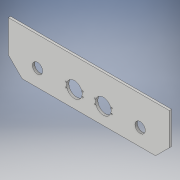
# Autodesk Inventor part: MecanumDriveTrainPlate17-18
Saved by Autodesk Inventor 2017 (Build 210142000, 142)
## iProperties
Created: 2017-09-16
Part Number: MecanumDriveTrainPlate17-18
Material: Generic
Document SubType Name: Modeling
Designer: User
Density: 1 g/cm^3
Appearance: Default
Author: User
Autodesk Inventor part; units mm, degrees
ref_plane "YZ Plane" through (0, 0, 0) normal (1, 0, 0) x (0, 1, 0)
ref_plane "XZ Plane" through (0, 0, 0) normal (0, 1, 0) x (-1, 0, 0)
ref_plane "XY Plane" through (0, 0, 0) normal (0, 0, 1) x (1, 0, 0)
sketch "Sketch1" plane through (0, 0, 0) normal (0, 0, 1) x (1, 0, 0)
  line L0 (0, 0) -> (444.5, 0)
  line L1 (444.5, 0) -> (444.5, 127)
  line L2 (444.5, 127) -> (0, 127)
  line L3 (0, 127) -> (0, 0)
  dimension "d0" = 444.5
  dimension "d1" = 127
  constraints: 8 end point, 2 perpendicular, 1 horizontal, 1 vertical
  measures "d0" distance of L0.start L0.end
  measures "d1" distance of L0.end L1.end
extrude "Extrusion1" add sketch "Sketch1" along normal blind 6.35
sketch "Sketch2" plane through (0, 0, 6.35) normal (0, 0, 1) x (1, 0, 0)
  line L0 (0, 0) -> (444.5, 0) projected
  line L1 (38.0923, 0) -> (0, 38.0919)
  line L2 (0, 127) -> (0, 0) projected
  line L3 (0, 0) -> (444.5, 0) projected
  line L4 (444.5, 0) -> (444.5, 127) projected
  line L5 (444.5, 0) -> (406.4, 0)
  line L6 (444.5, 0) -> (482.6, 0) construction
  line L7 (444.5, 0) -> (444.5, 38.0919)
  line L8 (444.5, 38.0919) -> (406.4086, 0)
  point P0 (419.1126, 0)
  dimension "d19" = 38.1
  dimension "d20" = 180
  constraints: 10 end point, 5 point on line, 3 collinear, 1 horizontal
  measures "d19" distance of L0.end L5.end
  measures "d20" angle of L5 L6
extrude "Extrusion2" cut sketch "Sketch2" against normal blind 50.8
sketch "Sketch3" plane through (0, 0, 6.35) normal (0, 0, 1) x (1, 0, 0)
  line L0 (0, 77.664) -> (80.645, 77.664) construction
  line L1 (444.5, 127) -> (0, 127) projected
  line L2 (80.645, 127) -> (161.29, 127) construction
  circle A0 centre (80.645, 46.355) radius 14.2748
  line L3 (444.5, 38.0919) -> (444.5, 127) projected
  line L4 (444.5, 77.664) -> (525.145, 77.664) construction
  line L5 (444.5, 38.0919) -> (444.5, 127) projected
  line L6 (444.5, 46.355) -> (525.145, 46.355) construction
  circle A1 centre (363.855, 46.355) radius 14.2748
  line L7 (444.5, 127) -> (0, 127) projected
  line L8 (0, 127) -> (0, 38.0919) projected
  circle A2 centre (182.245, 46.355) radius 21.59
  circle A3 centre (262.255, 46.355) radius 21.59
  line L9 (182.245, 46.355) -> (159.131, 46.355)
  line L10 (159.131, 46.355) -> (159.131, 53.3654)
  line L11 (159.131, 53.3654) -> (159.131, 46.355)
  line L12 (159.131, 46.355) -> (159.131, 39.3446)
  circle A4 centre (159.131, 39.3446) radius 1.7526
  circle A5 centre (159.131, 53.3654) radius 1.7526
  line L13 (182.245, 46.355) -> (205.359, 46.355)
  line L14 (205.359, 46.355) -> (205.359, 53.3654)
  line L15 (205.359, 53.3654) -> (205.359, 46.355)
  line L16 (205.359, 46.355) -> (205.359, 39.3446)
  circle A6 centre (205.359, 39.3446) radius 1.7526
  circle A7 centre (205.359, 53.3654) radius 1.7526
  line L17 (262.255, 46.355) -> (239.141, 46.355)
  line L18 (239.141, 46.355) -> (239.141, 53.3654)
  line L19 (239.141, 46.355) -> (239.141, 39.3446)
  circle A8 centre (239.141, 39.3446) radius 1.7526
  circle A9 centre (239.141, 53.3654) radius 1.7526
  line L20 (262.255, 46.355) -> (285.369, 46.355)
  line L21 (285.369, 46.355) -> (285.369, 39.3446)
  line L22 (285.369, 46.355) -> (285.369, 53.3654)
  circle A10 centre (285.369, 53.3654) radius 1.7526
  circle A11 centre (285.369, 39.3446) radius 1.7526
  point P0 (0, 0)
  dimension "d10" = 28.5496
  dimension "d18" = 28.5496
  dimension "d31" = 43.18
  dimension "d32" = 43.18
  dimension "d35" = 23.114
  dimension "d36" = 7.0104
  dimension "d37" = 7.0104
  dimension "d38" = 3.5052
  dimension "d39" = 3.5052
  dimension "d40" = 23.114
  dimension "d41" = 7.0104
  dimension "d42" = 7.0104
  dimension "d43" = 3.5052
  dimension "d44" = 3.5052
  dimension "d45" = 23.114
  dimension "d46" = 3.5052
  dimension "d47" = 3.5052
  dimension "d48" = 23.114
  dimension "d49" = 3.5052
  dimension "d50" = 3.5052
  constraints: 36 end point, 12 centre point, 8 coincident, 8 horizontal, 4 point on line, 4 vertical, 3 perpendicular, 2 collinear
  measures "d10" diameter of A0
  measures "d18" diameter of A1
  measures "d31" diameter of A2
  measures "d32" diameter of A3
  measures "d35" distance of L9.start L9.end
  measures "d36" distance of L9.end L10.end
  measures "d37" distance of L9.end L12.end
  measures "d38" diameter of A4
  measures "d39" diameter of A5
  measures "d40" distance of L9.start L13.end
  measures "d41" distance of L13.end L14.end
  measures "d42" distance of L13.end L16.end
  measures "d43" diameter of A6
  measures "d44" diameter of A7
  measures "d45" distance of L17.start L17.end
  measures "d46" diameter of A8
  measures "d47" diameter of A9
  measures "d48" distance of L17.start L20.end
  measures "d49" diameter of A10
  measures "d50" diameter of A11
extrude "Extrusion3" cut sketch "Sketch3" against normal blind 50.8 contours A0 | A1
extrude "Extrusion4" cut sketch "Sketch3" against normal blind 25.4 contours L13 L9 A2 | A2 L9 L13 | L20 L17 A3 | A3 L17 L20
extrude "Extrusion5" cut sketch "Sketch3" against normal blind 25.4 contours A4 | A5 | A6 | A7 | A8 | A9 | A10 | A11
body "Solid1"
